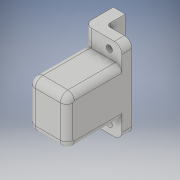
# Autodesk Inventor part: LockReciever
Saved by Autodesk Inventor 2019 (Build 230136000, 136)
## iProperties
Created: 2019-07-03
Part Number: LockReciever
Material: Generic
Document SubType Name: Modeling
Designer: garretthagen21
Density: 1 g/cm^3
Appearance: Default
Author: garretthagen21
Autodesk Inventor part; units mm, degrees
ref_plane "YZ Plane" through (0, 0, 0) normal (1, 0, 0) x (0, 1, 0)
ref_plane "XZ Plane" through (0, 0, 0) normal (0, 1, 0) x (-1, 0, 0)
ref_plane "XY Plane" through (0, 0, 0) normal (0, 0, 1) x (1, 0, 0)
sketch "Sketch2" plane through (0, 0, 0) normal (0, 0, 1) x (1, 0, 0)
  line L0 (-8.8906, 6.0836) -> (10.1594, 6.0836)
  line L1 (10.1594, 6.0836) -> (10.1594, -35.6994)
  line L2 (10.1594, -35.6994) -> (-8.8906, -35.6994)
  line L3 (-8.8906, -35.6994) -> (-8.8906, 6.0836)
  point P0 (0, 0)
  dimension "d2" = 19.05
  dimension "d3" = 41.783
  constraints: 8 end point, 2 parallel, 1 horizontal, 1 perpendicular
  measures "d2" distance of L1.end L2.end
  measures "d3" distance of L0.end L1.end
extrude "Extrusion1" add sketch "Sketch2" along normal blind 27.432
sketch "Sketch3" plane through (0, 0, 0) normal (0, 0, -1) x (-1, 0, 0)
  line L0 (-10.1594, 6.0836) -> (8.8906, 6.0836) projected
  line L1 (-10.1594, -35.6994) -> (-10.1594, 6.0836) projected
  line L2 (-10.1594, 6.0836) -> (2.7946, 6.0836)
  line L3 (2.7946, 6.0836) -> (2.7946, -35.6994)
  line L4 (2.7946, -35.6994) -> (-10.1594, -35.6994)
  line L5 (-10.1594, -35.6994) -> (-10.1594, 6.0836)
  dimension "d10" = 12.954
  dimension "d11" = 41.783
  constraints: 8 end point, 2 parallel, 1 horizontal, 1 perpendicular
  measures "d10" distance of L3.end L4.end
  measures "d11" distance of L2.end L3.end
extrude "Extrusion2" cut sketch "Sketch3" against normal blind 9.652
sketch "Sketch4" plane through (0, 0, 27.432) normal (0, 0, 1) x (1, 0, 0)
  line L0 (-8.8906, 6.0836) -> (-8.8906, -35.6994) projected
  line L1 (10.1594, -35.6994) -> (10.1594, 6.0836) projected
  line L2 (-8.8906, 6.0836) -> (10.1594, 6.0836)
  line L3 (10.1594, 6.0836) -> (10.1594, -2.8064)
  line L4 (10.1594, -2.8064) -> (-8.8906, -2.8064)
  line L5 (-8.8906, -2.8064) -> (-8.8906, 6.0836)
  line L6 (10.1594, -35.6994) -> (-8.8906, -35.6994)
  line L7 (-8.8906, -35.6994) -> (-8.8906, -26.8094)
  line L8 (-8.8906, -26.8094) -> (10.1594, -26.8094)
  line L9 (10.1594, -26.8094) -> (10.1594, -35.6994)
  point P0 (0, 0)
  dimension "d12" = 8.89
  dimension "d13" = 8.89
  constraints: 16 end point, 4 parallel, 2 horizontal, 2 perpendicular, 2 point on line
  measures "d12" distance of L2.end L3.end
  measures "d13" distance of L6.end L7.end
extrude "Extrusion3" cut sketch "Sketch4" against normal blind 12.7 contours L2 L1 L4 L0 | L8 L1 L6 L0
sketch "Sketch6" plane through (0, 0, 27.432) normal (0, 0, 1) x (1, 0, 0)
  line L0 (10.1594, -26.8094) -> (10.1594, -2.8064) projected
  line L1 (-8.8906, -2.8064) -> (-8.8906, -26.8094) projected
  line L2 (10.1594, -26.8094) -> (-8.8906, -26.8094)
  line L3 (-8.8906, -26.8094) -> (-8.8906, -2.8064)
  line L4 (-8.8906, -2.8064) -> (10.1594, -2.8064)
  line L5 (10.1594, -2.8064) -> (10.1594, -26.8094)
  point P0 (0, 0)
  constraints: 8 end point, 2 parallel, 1 horizontal, 1 perpendicular
extrude "Extrusion4" add sketch "Sketch6" along normal blind 15.24
sketch "Sketch8" plane through (-8.8906, -35.6994, 0) normal (-1, 0, 0) x (0, 0, 1)
  line L0 (42.672, 32.893) -> (14.732, 32.893) projected
  line L1 (42.672, 32.893) -> (42.672, 8.89) projected
  line L2 (14.732, 8.89) -> (42.672, 8.89) projected
  line L3 (20.32, 20.8915) -> (20.32, 14.478)
  line L4 (20.32, 14.478) -> (37.084, 14.478)
  line L5 (37.084, 14.478) -> (37.084, 27.305)
  line L6 (37.084, 27.305) -> (20.32, 27.305)
  line L7 (20.32, 27.305) -> (20.32, 20.8915)
  point P0 (0, 35.6994)
  constraints: 10 end point, 4 perpendicular, 1 point on line, 1 vertical
extrude "Extrusion5" cut sketch "Sketch8" against normal blind 15.24
sketch "Sketch9" plane through (0, 0, 14.732) normal (0, 0, 1) x (1, 0, 0)
  line L0 (10.1594, -26.8094) -> (10.1594, -35.6994) projected
  line L1 (10.1594, -35.6994) -> (-8.8906, -35.6994) projected
  line L2 (-8.8906, 6.0836) -> (10.1594, 6.0836) projected
  line L3 (10.1594, 6.0836) -> (10.1594, -2.8064) projected
  point P0 (0, 0)
  point P1 (3.8094, 1.6386)
  point P2 (3.8094, -31.2544)
  dimension "d29" = 6.35
  dimension "d30" = 4.445
  dimension "d31" = 4.445
  dimension "d32" = 6.35
  measures "d29" distance from line of point (3.809, -31.254) L0
  measures "d30" distance from line of point (3.809, -31.254) L1
  measures "d31" distance from line of point (3.809, 1.639) L2
  measures "d32" distance from line of point (3.809, 1.639) L3
hole "Hole1" at (3.8094, -31.2544, 14.732) at (3.8094, 1.6386, 14.732) direction (0, 0, -1) diameter 3.175 end through all
sketch "Sketch10" plane through (-8.8906, -35.6994, 0) normal (-1, 0, 0) x (0, 0, 1)
  line L0 (0, 0) -> (0, 41.783) projected
  line L1 (42.672, 32.893) -> (14.732, 32.893) projected
  line L2 (14.732, 8.89) -> (42.672, 8.89) projected
  point P0 (0, 35.6994)
  point P1 (4.826, 24.892)
  point P2 (4.826, 16.891)
  dimension "d40" = 4.826
  dimension "d41" = 4.826
  dimension "d42" = 8.001
  dimension "d43" = 8.001
  measures "d40" distance from line of point (4.826, 24.892) L0
  measures "d41" distance from line of L0 point (4.826, 16.891)
  measures "d42" distance from line of point (4.826, 24.892) L1
  measures "d43" distance from line of point (4.826, 16.891) L2
hole "Hole2" at (-8.8906, -10.8074, 4.826) at (-8.8906, -18.8084, 4.826) direction (1, 0, 0) diameter 3.175 end through all counterbore diameter 6.223 counterbore depth 1.905
fillet "Fillet1" radius 3.81 6 edges at (-8.8906, -31.2544, 14.732) (0.6344, -26.8094, 42.672) (10.1594, -35.6994, 12.192) (10.1594, 6.0836, 12.192) (0.6344, -2.8064, 42.672) (-8.8906, 1.6386, 14.732)
fillet "Fillet2" radius 1.905 1 edges at (-2.7946, -14.8079, 9.652)
fillet "Fillet3" radius 3.175 12 edges at (-8.8906, -25.6935, 41.5561) (-8.8906, -14.8079, 42.672) (-8.8906, -3.9224, 41.5561) (-8.8906, -2.8064, 26.797) (-8.8906, -2.8064, 12.827) (-8.8906, -26.8094, 26.797) (-8.8906, -26.8094, 12.827) (10.1594, -25.6935, 41.5561) (10.1594, -14.8079, 42.672) (10.1594, -3.9224, 41.5561) (10.1594, -2.8064, 26.797) (10.1594, -26.8094, 26.797)
body "Solid1"
